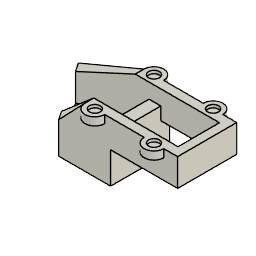
colour_detection_mechanism (Autodesk Fusion 360 archive; units mm, degrees)
design "Colour Sensor Holder"
part number: 2025-08-24-10-22-08-973
Autodesk Fusion 360 part; units mm, degrees
sketch "Base" plane through (0, 0, 0) normal (0, 0, 1) x (1, 0, 0)
  line L0 (0, 0) -> (46.334, 0)
  line L1 (46.334, 0) -> (46.334, 30)
  line L2 (46.334, 30) -> (0, 30)
  line L3 (0, 30) -> (0, 0)
  dimension "d2" = 46.334
  dimension "d3" = 30
  constraint horizontal L0
  constraint vertical L1
  constraint horizontal L2
  constraint vertical L3
  constraint coincident L0.start L3.end
  measures "d2" distance of L0.start L0.end
  measures "d3" distance of L0.end L1.end
extrude "Extrude1" add sketch "Base" along normal blind 4
sketch "Side Profile" plane through (0, 0, 0) normal (0, -1, 0) x (1, 0, 0)
  line L0 (0, 0) -> (46.334, 0)
  line L1 (46.334, 0) -> (46.334, 4)
  line L2 (46.334, 4) -> (0, 4)
  line L3 (0, 4) -> (0, 0)
  line L4 (46.334, 4) -> (46.334, 16)
  line L5 (46.334, 16) -> (80.334, 16)
  line L6 (80.334, 16) -> (80.334, 30)
  line L7 (80.334, 30) -> (0, 30)
  line L8 (0, 30) -> (0, 4)
  dimension "d6" = 12
  dimension "d7" = 34
  dimension "d8" = 14
  dimension "d11" = 46.334
  dimension "d52" = 80.334
  constraint coincident L1.end L2.start
  constraint perpendicular L2 L4
  constraint perpendicular L4 L5
  constraint perpendicular L5 L6
  constraint perpendicular L6 L7
  constraint coincident L2.end L3.start
  constraint perpendicular L2 L8
  measures "d6" distance of L1.end L4.end
  measures "d7" distance of L4.end L5.end
  measures "d8" distance of L5.end L6.end
  measures "d11" distance of L0.start L0.end
  measures "d52" distance of L6.end L7.end
extrude "Extrude2" add sketch "Side Profile" against normal blind 4.5 contours L2 L4 L5 L6 L7 L8
extrude "Extrude3" add sketch "Side Profile" against normal blind 4.5 from surface at -25.5 contours L2 L4 L5 L6 L7 L8
sketch "Front End" plane through (0, 0, 0) normal (0, -1, 0) x (1, 0, 0)
  line L0 (0, 0) -> (46.334, 0)
  line L1 (46.334, 0) -> (46.334, 16)
  line L2 (46.334, 16) -> (80.334, 16)
  line L3 (80.334, 16) -> (80.334, 30)
  line L4 (80.334, 30) -> (0, 30)
  line L5 (0, 30) -> (0, 0)
  line L6 (80.334, 30) -> (76.034, 30)
  line L7 (76.034, 30) -> (76.034, 16)
  line L8 (76.034, 16) -> (80.334, 16)
  line L9 (80.334, 16) -> (80.334, 30)
  dimension "d17" = 4.3
  constraint horizontal L6
  constraint vertical L7
  constraint horizontal L8
  constraint vertical L9
  constraint coincident L3.end L4.start
  constraint collinear L2 L8
  measures "d17" distance of L3.end L6.end
extrude "Extrude4" add sketch "Front End" against normal blind 30 contours L2 L3 L4 L6 L7 L8 L9
sketch "Middle End" plane through (0, 0, 0) normal (0, -1, 0) x (1, 0, 0)
  line L0 (80.334, 30) -> (0, 30)
  line L1 (0, 30) -> (0, 0)
  line L2 (0, 0) -> (46.334, 0)
  line L3 (46.334, 0) -> (46.334, 16)
  line L4 (46.334, 16) -> (80.334, 16)
  line L5 (80.334, 16) -> (80.334, 30)
  line L6 (46.334, 22.5) -> (40.334, 22.5)
  line L7 (40.334, 22.5) -> (40.334, 0)
  line L8 (40.334, 0) -> (46.334, 0)
  line L9 (46.334, 0) -> (46.334, 22.5)
  dimension "d20" = 7.5
  dimension "d21" = 6
  constraint horizontal L6
  constraint vertical L7
  constraint horizontal L8
  constraint vertical L9
  constraint collinear L3 L9
  constraint collinear L2 L8
  measures "d20" distance of L0 L6
  measures "d21" distance of L6.start L6.end
extrude "Extrude5" add sketch "Middle End" against normal blind 30 contours L2 L3 L6 L7 L8 L9
sketch "Lip" plane through (76.034, 0, 0) normal (-1, 0, 0) x (0, -1, 0)
  line L0 (-25.5, 30) -> (-25.5, 16)
  line L1 (-25.5, 16) -> (-4.5, 16)
  line L2 (-4.5, 16) -> (-4.5, 30)
  line L3 (-4.5, 30) -> (-25.5, 30)
  line L4 (-18, 25) -> (-12, 25)
  line L5 (-12, 25) -> (-12, 21)
  line L6 (-12, 21) -> (-18, 21)
  line L7 (-18, 21) -> (-18, 25)
  dimension "d24" = 5
  dimension "d25" = 6
  dimension "d26" = 4
  dimension "d27" = 7.5
  constraint horizontal L4
  constraint vertical L5
  constraint horizontal L6
  constraint vertical L7
  measures "d24" distance of L3 L4
  measures "d25" distance of L4.start L4.end
  measures "d26" distance of L4.start L6.end
  measures "d27" distance of L0 L7
extrude "Extrude6" add sketch "Lip" along normal blind 4 contours L4 L5 L6 L7
sketch "Magnet Holders" plane through (0, 0, 30) normal (0, 0, 1) x (-1, 0, 0)
  line L0 (-80.334, -30) -> (0, -30)
  line L1 (0, -30) -> (0, -25.5)
  line L2 (0, -25.5) -> (-76.034, -25.5)
  line L3 (-76.034, -25.5) -> (-76.034, -4.5)
  line L4 (-76.034, -4.5) -> (0, -4.5)
  line L5 (0, -4.5) -> (0, 0)
  line L6 (0, 0) -> (-80.334, 0)
  line L7 (-80.334, 0) -> (-80.334, -30)
  circle A0 centre (-68.334, -30) radius 5
  circle A1 centre (-38.334, -30) radius 5
  circle A2 centre (-38.334, 0) radius 5
  circle A3 centre (-68.334, 0) radius 5
  circle A4 centre (-38.334, 0) radius 2.75
  circle A5 centre (-68.334, 0) radius 2.75
  circle A6 centre (-38.334, -30) radius 2.75
  circle A7 centre (-68.334, -30) radius 2.75
  dimension "d33" = 10
  dimension "d34" = 10
  dimension "d35" = 10
  dimension "d36" = 10
  dimension "d37" = 12
  dimension "d38" = 12
  dimension "d43" = 5.5
  dimension "d44" = 5.5
  dimension "d45" = 5.5
  dimension "d46" = 5.5
  dimension "d50" = 42
  dimension "d51" = 42
  constraint coincident L0 A0.centre
  constraint coincident L0 A1.centre
  constraint coincident L6 A2.centre
  constraint coincident L6 A3.centre
  constraint concentric A2 A4
  constraint concentric A3 A5
  constraint concentric A1 A6
  constraint concentric A0 A7
  measures "d33" diameter of A0
  measures "d34" diameter of A1
  measures "d35" diameter of A2
  measures "d36" diameter of A3
  measures "d37" distance of L6.end A3.centre
  measures "d38" distance of L0.start A0.centre
  measures "d43" diameter of A4
  measures "d44" diameter of A5
  measures "d45" diameter of A6
  measures "d46" diameter of A7
  measures "d50" distance of L0.start A1.centre
  measures "d51" distance of L6.end A2.centre
extrude "Extrude8" add sketch "Magnet Holders" against normal blind 4 contours L0 A7 | L0 A0 A7 | L0 A1 A6 | L0 A6 | L6 A3 A5 | L6 A5 | L6 A2 A4 | L6 A4 picked at (-68.2655, -30.9141) picked at (-37.4674, -30.6679) picked at (-68.2655, 0.9141) picked at (-39.0365, 1.0303)
extrude "Extrude9" cut sketch "Magnet Holders" against normal blind 1.5 contours L0 A7 | L0 A7 | L0 A6 | L0 A6 | L6 A5 | L6 A5 | L6 A4 | L6 A4
sketch "Conduit Angle" plane through (0, 0, 30) normal (0, 0, 1) x (-1, 0, 0)
  circle A0 centre (-68.334, 0) radius 2.75
  circle A1 centre (-38.334, -30) radius 2.75
  circle A2 centre (-38.334, 0) radius 2.75
  circle A3 centre (-68.334, -30) radius 2.75
  line L0 (-33.334, -30) -> (0, -30)
  line L1 (0, -30) -> (0, -25.5)
  line L2 (0, -25.5) -> (-76.034, -25.5)
  line L3 (-76.034, -25.5) -> (-76.034, -4.5)
  line L4 (-76.034, -4.5) -> (0, -4.5)
  line L5 (0, -4.5) -> (0, 0)
  line L6 (0, 0) -> (-33.334, 0)
  arc A4 (-33.334, 0) -> (-43.334, 0) centre (-38.334, 0) ccw
  line L7 (-43.334, 0) -> (-63.334, 0)
  arc A5 (-63.334, 0) -> (-73.334, 0) centre (-68.334, 0) ccw
  line L8 (-73.334, 0) -> (-80.334, 0)
  line L9 (-80.334, 0) -> (-80.334, -30)
  line L10 (-80.334, -30) -> (-73.334, -30)
  arc A6 (-73.334, -30) -> (-63.334, -30) centre (-68.334, -30) ccw
  line L11 (-63.334, -30) -> (-43.334, -30)
  arc A7 (-43.334, -30) -> (-33.334, -30) centre (-38.334, -30) ccw
  line L12 (-40.334, -4.5) -> (-40.334, -25.5)
  line L13 (-40.334, -25.5) -> (0, -25.5)
  line L14 (0, -25.5) -> (0, -4.5)
  line L15 (0, -4.5) -> (-40.334, -4.5)
  line L16 (0, -30) -> (-19.932, 0)
  dimension "d53" = 33.6
  constraint coincident L0.end L1.start
  constraint coincident L6 L16.end
  measures "d53" angle of L14 L16
extrude "Extrude10" cut sketch "Conduit Angle" against normal blind 30 contours L1 L2 L13 L16 | L2 L4 L13 L14 L15 L16 | L4 L5 L6 L15 L16
sketch "Conduit Height" plane through (13.8279, 9.1873, 0) normal (-0.832921, -0.553392, 0) x (0.553392, -0.832921, 0)
  line L0 (-19.585, 4) -> (-19.585, 30)
  line L1 (-19.585, 30) -> (-24.9876, 30)
  line L2 (-24.9876, 30) -> (-24.9876, 0)
  line L3 (-24.9876, 0) -> (11.0302, 0)
  line L4 (11.0302, 0) -> (11.0302, 30)
  line L5 (11.0302, 30) -> (5.6275, 30)
  line L6 (5.6275, 30) -> (5.6275, 4)
  line L7 (5.6275, 4) -> (-19.585, 4)
  line L8 (-24.9876, 0) -> (11.0302, 0)
  line L9 (11.0302, 0) -> (11.0302, 16)
  line L10 (11.0302, 16) -> (-24.9876, 16)
  line L11 (-24.9876, 16) -> (-24.9876, 0)
  point P0 (5.6275, 16)
  point P1 (-19.585, 16)
  dimension "d56" = 16
  constraint horizontal L8
  constraint vertical L9
  constraint horizontal L10
  constraint vertical L11
  constraint coincident L4 L9.end
  constraint coincident L2.end L3.start
  constraint coincident L10 P0
  constraint coincident L6 P0
  constraint coincident L10 P1
  constraint coincident L0 P1
  measures "d56" distance of L8 L10
sketch "Colour Sensor Cover Shape" plane through (0, 0, 30) normal (0, 0, 1) x (-1, 0, 0)
  line L0 (0, -30) -> (-2.9898, -25.5)
  line L1 (-2.9898, -25.5) -> (-76.034, -25.5)
  line L2 (-76.034, -25.5) -> (-76.034, -4.5)
  line L3 (-76.034, -4.5) -> (-16.9422, -4.5)
  line L4 (-16.9422, -4.5) -> (-19.932, 0)
  line L5 (-19.932, 0) -> (-33.334, 0)
  arc A0 (-33.334, 0) -> (-43.334, 0) centre (-38.334, 0) ccw
  line L6 (-43.334, 0) -> (-63.334, 0)
  arc A1 (-63.334, 0) -> (-73.334, 0) centre (-68.334, 0) ccw
  line L7 (-73.334, 0) -> (-80.334, 0)
  line L8 (-80.334, 0) -> (-80.334, -30)
  line L9 (-80.334, -30) -> (-73.334, -30)
  arc A2 (-73.334, -30) -> (-63.334, -30) centre (-68.334, -30) ccw
  line L10 (-63.334, -30) -> (-43.334, -30)
  arc A3 (-43.334, -30) -> (-33.334, -30) centre (-38.334, -30) ccw
  line L11 (-33.334, -30) -> (0, -30)
  circle A4 centre (-68.334, 0) radius 2.75
  circle A5 centre (-38.334, -30) radius 2.75
  circle A6 centre (-38.334, 0) radius 2.75
  circle A7 centre (-68.334, -30) radius 2.75
  line L12 (-33.334, -30) -> (-33.334, 0)
  point P0 (-33.334, -25.5)
  point P1 (-33.334, -4.5)
  constraint coincident A3.end L11.start
  constraint coincident L5.end A0.start
  constraint coincident L1 P0
  constraint coincident L12 P0
  constraint coincident L3 P1
  constraint coincident L12 P1
sketch "Right Loft Outside Shape" plane through (0, 0, 0) normal (0, -1, 0) x (1, 0, 0)
  line L0 (19.932, 30) -> (19.932, 0)
  line L1 (19.932, 0) -> (46.334, 0)
  line L2 (46.334, 0) -> (46.334, 16)
  line L3 (46.334, 16) -> (80.334, 16)
  line L4 (80.334, 16) -> (80.334, 30)
  line L5 (80.334, 30) -> (73.334, 30)
  line L6 (73.334, 30) -> (73.334, 26)
  line L7 (73.334, 26) -> (63.334, 26)
  line L8 (63.334, 26) -> (63.334, 30)
  line L9 (63.334, 30) -> (43.334, 30)
  line L10 (43.334, 30) -> (43.334, 26)
  line L11 (43.334, 26) -> (33.334, 26)
  line L12 (33.334, 26) -> (33.334, 30)
  line L13 (33.334, 30) -> (19.932, 30)
  line L14 (33.334, 30) -> (19.932, 16)
  point P0 (33.334, 30)
  point P1 (19.932, 16)
  constraint coincident P0 L12.end
  constraint coincident P1 L14.end
sketch "Right Loft Inside Shape" plane through (0, 4.5, 0) normal (0, 1, 0) x (-1, 0, 0)
  line L0 (-16.9422, 4) -> (-16.9422, 30)
  line L1 (-16.9422, 30) -> (-76.034, 30)
  line L2 (-76.034, 30) -> (-76.034, 16)
  line L3 (-76.034, 16) -> (-46.334, 16)
  line L4 (-46.334, 16) -> (-46.334, 22.5)
  line L5 (-46.334, 22.5) -> (-40.334, 22.5)
  line L6 (-40.334, 22.5) -> (-40.334, 4)
  line L7 (-40.334, 4) -> (-16.9422, 4)
  line L8 (-33.334, 30) -> (-16.9422, 16)
  point P0 (-33.334, 30)
  point P1 (-16.9422, 16)
  constraint coincident P0 L8.start
  constraint coincident P1 L8.end
sketch "Left Loft Inside Shape" plane through (0, 25.5, 0) normal (0, -1, 0) x (1, 0, 0)
  line L0 (2.9898, 30) -> (2.9898, 4)
  line L1 (2.9898, 4) -> (40.334, 4)
  line L2 (40.334, 4) -> (40.334, 22.5)
  line L3 (40.334, 22.5) -> (46.334, 22.5)
  line L4 (46.334, 22.5) -> (46.334, 16)
  line L5 (46.334, 16) -> (76.034, 16)
  line L6 (76.034, 16) -> (76.034, 30)
  line L7 (76.034, 30) -> (2.9898, 30)
  line L8 (33.334, 30) -> (2.9898, 16)
  point P0 (33.334, 30)
  point P1 (2.9898, 16)
  constraint coincident P0 L8.start
  constraint coincident P1 L8.end
sketch "Left Loft Outside Shape" plane through (0, 30, 0) normal (0, 1, 0) x (-1, 0, 0)
  line L0 (-33.334, 30) -> (-33.334, 26)
  line L1 (-33.334, 26) -> (-43.334, 26)
  line L2 (-43.334, 26) -> (-43.334, 30)
  line L3 (-43.334, 30) -> (-63.334, 30)
  line L4 (-63.334, 30) -> (-63.334, 26)
  line L5 (-63.334, 26) -> (-73.334, 26)
  line L6 (-73.334, 26) -> (-73.334, 30)
  line L7 (-73.334, 30) -> (-80.334, 30)
  line L8 (-80.334, 30) -> (-80.334, 16)
  line L9 (-80.334, 16) -> (-46.334, 16)
  line L10 (-46.334, 16) -> (-46.334, 0)
  line L11 (-46.334, 0) -> (0, 0)
  line L12 (0, 0) -> (0, 30)
  line L13 (0, 30) -> (-33.334, 30)
  line L14 (-33.334, 30) -> (0, 16)
  point P0 (-33.334, 30)
  point P1 (0, 16)
  constraint coincident P0 L0.start
  constraint coincident P1 L14.end
loft "Loft1" cut profiles "Right Loft Outside Shape", "Right Loft Inside Shape" section 1 contours L0 L13 L14 section 2 contours L0 L1 L8
loft "Loft2" cut profiles "Left Loft Inside Shape", "Left Loft Outside Shape" section 1 contours L0 L7 L8 section 2 contours L12 L13 L14
chamfer "Chamfer2" distance 4 distance2 2 1 edges at (9.966, 15, 4) measured on face at (20.0887, 18.5, 4)
equation "base_plate_thickness = 4 mm" comment "Thickness of the Colour Detection Mechanism Platform's base plate."
equation "d4 = base_plate_thickness"
equation "d37 = 7 mm + 5 mm"
equation "d38 = 7 mm + 5 mm"
named bodies: "Colour Sensor Holder"

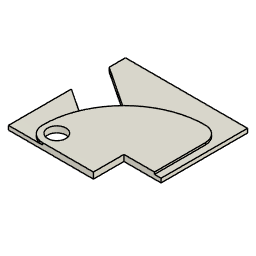
design "Colour Detection Mechanism Platform"
Autodesk Fusion 360 part; units mm, degrees
sketch "Colour Detection Mechanism Platform" plane through (0, 0, 0) normal (0, 0, 1) x (1, 0, 0)
  line L0 (0, 0) -> (120, 0)
  line L1 (120, 0) -> (120, 76)
  line L2 (120, 76) -> (0, 76)
  line L3 (0, 76) -> (0, 0)
  dimension "d169" = 120
  dimension "d170" = 76
  constraint horizontal L0
  constraint vertical L1
  constraint horizontal L2
  constraint vertical L3
  constraint coincident L0.start L3.end
  measures "d169" distance of L0.start L0.end
  measures "d170" distance of L0.start L2.end
extrude "Extrude42" add sketch "Colour Detection Mechanism Platform" along normal blind 4
sketch "Smartie Path" plane through (0, 0, 4) normal (0, 0, 1) x (-1, 0, 0)
  line L0 (0, -76) -> (0, 0)
  line L1 (0, 0) -> (-120, 0)
  line L2 (-120, 0) -> (-120, -76)
  line L3 (-120, -76) -> (0, -76)
  circle A0 centre (-98.5, 24) radius 80
  line L4 (-98.5, 24) -> (-113.5, 24)
  line L5 (-113.5, 24) -> (-113.5, -56)
  line L6 (-113.5, -56) -> (-98.5, -56)
  line L7 (-98.5, -56) -> (-98.5, 24)
  line L8 (-98.5, 24) -> (-18.5, 24)
  line L9 (-18.5, 24) -> (-18.5, 39)
  line L10 (-18.5, 39) -> (-98.5, 39)
  line L11 (-98.5, 39) -> (-98.5, 24)
  line L12 (-98.5, 24) -> (-113.5, 24)
  line L13 (-113.5, 24) -> (-113.5, 39)
  line L14 (-113.5, 39) -> (-98.5, 39)
  line L15 (-98.5, 39) -> (-98.5, 24)
  circle A1 centre (-32.5, 24) radius 9
  dimension "d173" = 160
  dimension "d174" = 24
  dimension "d175" = 21.5
  dimension "d176" = 15
  dimension "d177" = 15
  dimension "d178" = 80
  dimension "d179" = 80
  dimension "d184" = 18
  dimension "d185" = 14
  constraint horizontal L4
  constraint vertical L5
  constraint horizontal L6
  constraint vertical L7
  constraint coincident A0.centre L4.start
  constraint horizontal L8
  constraint vertical L9
  constraint horizontal L10
  constraint vertical L11
  constraint horizontal L12
  constraint vertical L13
  constraint horizontal L14
  constraint vertical L15
  constraint collinear L5 L13
  constraint collinear L10 L14
  constraint coincident L8 A1.centre
  measures "d173" diameter of A0
  measures "d174" distance of L1 A0.centre
  measures "d175" horizontal distance of L1.end A0.centre
  measures "d176" distance of L8.end L9.end
  measures "d177" distance of L5.end L6.end
  measures "d178" distance of L4.end L5.end
  measures "d179" distance of L9.end L10.end
  measures "d184" diameter of A1
  measures "d185" distance of L8.end A1.centre
extrude "Extrude43" add sketch "Smartie Path" along normal blind 2 contours L1 A0 L7 | L1 A0 L7 L8 A1 | L1 A0 L5 L7 | L1 L4 L5 L7 L12 | A0 L8 L10 L11 L15 A1 | L4 L11 L12 L13 L14 L15
fillet "Fillet2" radius 15 2 edges at (19.9188, -39, 5) (113.5, 54.5812, 5)
extrude "Extrude44" add 1 faces at (89.4665, -20.5529, 4) along direction (0, 0, -1) blind 4
sketch "Servo Hole" plane through (0, 0, 6) normal (0, 0, 1) x (-1, 0, 0)
  circle A0 centre (-32.5, 24) radius 9
  arc A1 (-113.5, -41) -> (-98.5, -56) centre (-98.5, -41) ccw
  arc A2 (-98.5, -56) -> (-18.5, 24) centre (-98.5, 24) ccw
  arc A3 (-18.5, 24) -> (-33.5, 39) centre (-33.5, 24) ccw
  line L0 (-33.5, 39) -> (-113.5, 39)
  line L1 (-113.5, 39) -> (-113.5, -41)
  line L2 (-113.5, 39) -> (-83.5, 39)
  line L3 (-83.5, 39) -> (-83.5, 9)
  line L4 (-83.5, 9) -> (-113.5, 9)
  line L5 (-113.5, 9) -> (-113.5, 39)
  dimension "d188" = 30
  dimension "d189" = 30
  constraint horizontal L2
  constraint vertical L3
  constraint horizontal L4
  constraint vertical L5
  constraint coincident L0.end L1.start
  measures "d188" distance of L3.end L4.end
  measures "d189" distance of L2.end L3.end
extrude "Extrude45" cut sketch "Servo Hole" against normal blind 6 contours L0 L1 L2 L3 L4 L5
sketch "Colour Sensor Holder Hole" plane through (0, 0, 4) normal (0, 0, 1) x (-1, 0, 0)
  line L0 (-120, 0) -> (-120, -76)
  line L1 (-120, -76) -> (0, -76)
  line L2 (0, -76) -> (0, 0)
  line L3 (-113.5, 0) -> (-120, 0)
  arc A0 (-98.5, -56) -> (-22.1849, 0) centre (-98.5, 24) ccw
  arc A1 (-113.5, -41) -> (-98.5, -56) centre (-98.5, -41) ccw
  line L4 (-113.5, -41) -> (-113.5, 0)
  line L5 (0, -59.401) -> (-38.732, -33.6675)
  line L6 (0, -23.4021) -> (-22.139, -8.693)
  line L7 (-38.732, -33.6675) -> (-22.139, -8.693)
  line L8 (0, -60.0013) -> (-39.4252, -33.8073)
  line L9 (-39.4252, -33.8073) -> (-22.2788, -7.9998)
  line L10 (-22.2788, -7.9998) -> (0, -22.8018)
  line L11 (0, 0) -> (-22.1849, 0)
  dimension "d249" = 56.4
  dimension "d250" = 59.401
  dimension "d254" = 56.4
  dimension "d255" = 8.693
  dimension "d256" = 22.139
  dimension "d257" = 23.4021
  dimension "d258" = 38.732
  dimension "d261" = 0.5
  dimension "d262" = 0.5
  dimension "d263" = 0.5
  constraint coincident L2 L5.start
  constraint coincident L2 L6.start
  constraint coincident L2 L8.start
  constraint coincident L2 L10.end
  constraint perpendicular L9 L10
  constraint parallel L5 L8
  constraint parallel L7 L9
  measures "d249" angle of L2 L5
  measures "d250" distance of L2.end L5.start
  measures "d254" angle of L2 L6
  measures "d255" distance of L3 L6.end
  measures "d256" horizontal distance of L2.end L6.end
  measures "d257" distance of L2.end L6.start
  measures "d258" horizontal distance of L5.start L5.end
  measures "d261" distance of L5 L8
  measures "d262" distance of L7 L9
extrude "Extrude58" cut sketch "Colour Sensor Holder Hole" against normal blind 4 contours L2 L5 L6 L7
extrude "Extrude59" cut sketch "Colour Sensor Holder Hole" against normal blind 4 contours L2 L5 L6 L7 L8 L9 L10
sketch "Platform Extension" plane through (0, 0, 4) normal (0, 0, 1) x (-1, 0, 0)
  line L0 (-22.2788, -7.9998) -> (0, -22.8018)
  line L1 (0, -22.8018) -> (0, 0)
  line L2 (0, 0) -> (-22.1849, 0)
  arc A0 (-98.5, -56) -> (-22.1849, 0) centre (-98.5, 24) ccw
  arc A1 (-113.5, -41) -> (-98.5, -56) centre (-98.5, -41) ccw
  line L3 (-113.5, -41) -> (-113.5, 0)
  line L4 (-120, 0) -> (-120, -76)
  line L5 (-120, -76) -> (0, -76)
  line L6 (0, -60.0013) -> (-39.4252, -33.8073)
  line L7 (-39.4252, -33.8073) -> (-22.2788, -7.9998)
  line L8 (-83.5, 9) -> (-113.5, 9)
  line L9 (-113.5, 9) -> (-113.5, -41)
  arc A2 (-113.5, -41) -> (-98.5, -56) centre (-98.5, -41) ccw
  arc A3 (-98.5, -56) -> (-18.5, 24) centre (-98.5, 24) ccw
  arc A4 (-18.5, 24) -> (-33.5, 39) centre (-33.5, 24) ccw
  line L10 (-33.5, 39) -> (-83.5, 39)
  line L11 (-83.5, 39) -> (-83.5, 9)
  circle A5 centre (-32.5, 24) radius 9
  line L12 (0, 0) -> (0, 39)
  line L13 (0, 39) -> (-33.5, 39)
  line L14 (-113.5, 0) -> (-120, 0)
  line L15 (0, -76) -> (0, -60.0013)
  line L16 (-113.5, 0) -> (-120, 0)
  line L17 (-120, 0) -> (-120, 9)
  line L18 (-120, 9) -> (-113.5, 9)
  line L19 (-113.5, 9) -> (-113.5, 0)
  constraint coincident L1.end L2.start
  constraint coincident A4.end L10.start
  constraint perpendicular L2 L12
  constraint perpendicular L12 L13
  constraint horizontal L16
  constraint vertical L17
  constraint horizontal L18
  constraint vertical L19
  constraint coincident L3.end L14.start
  constraint collinear L4 L17
  constraint collinear L8 L18
extrude "Extrude60" add sketch "Platform Extension" against normal blind 4 contours L2 A3 A4 L12 L13 | L9 L14 L16 L17 L18 L19
equation "d95 = 4 mm + 1.5 mm"
equation "d103 = -( 29 mm - 16 mm )"
named bodies: "Colour Detection Mechanism Platform"
